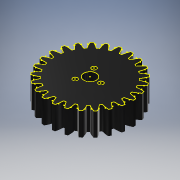
# Autodesk Inventor part: Spur Gear2
Saved by Autodesk Inventor 2017 (Build 210142000, 142)
## iProperties
Created: 2018-10-18
Part Number: Spur Gear2
Material: ABS Plastic
Document SubType Name: Modeling
Designer: Dell
Categories: <?xml version="1.0" encoding="UTF-16"?> <MemberInstance><Categories><FamilyTemplate><FamilyTemplateParameter ValueType="xs:double" Id="1" ObjectReferenceKey="da_z" ObjectType="kUserParameterObject"/><FamilyTemplateParameter ValueType="xs:double" Id="2" ObjectReferenceKey="da_b" ObjectType="kUserParameterObject"/><FamilyTemplateParameter ValueType="xs:double" Id="3" ObjectReferenceKey="da_beta" ObjectType="kUserParameterObject"/><FamilyTemplateParameter ValueType="xs:double" Id="4" ObjectReferenceKey="da_da" ObjectType="kUserParameterObject"/><FamilyTemplateParameter ValueType="xs:double" Id="5" ObjectReferenceKey="da_aw" ObjectType="kUserParameterObject"/><FamilyTemplateParameter ValueType="xs:string" Id="6" ObjectReferenceKey="EAIAABAAAACIAQAAAAAAAIAAAAAAAAAA" ObjectType="83910656" SubObjectId="SurfaceGeometry"/></FamilyTemplate><ParamToTemplateMap><ParamToTemplate CategoryParameter="//CategoryParameter[@InternalName='046C89C9-8512-4d59-83FE-43B91F4F132A']" TemplateParameter="1"/><ParamToTemplate CategoryParameter="//CategoryParameter[@InternalName='2552DF32-E462-4b46-AEBF-C6C7768E72AC']" TemplateParameter="2"/><ParamToTemplate CategoryParameter="//CategoryParameter[@InternalName='C9EE641D-15FC-4fae-A226-E94C4372FDD7']" TemplateParameter="3"/><ParamToTemplate><ParamToTemplate CategoryParameter="//CategoryParameter[@InternalName='00B6519A-459B-49c7-AD84-2E56D39A5744']" ConstantValue="0.000000"/></ParamToTemplate><ParamToTemplate><ParamToTemplate CategoryParameter="//CategoryParameter[@InternalName='04B31F0E-C7A6-4894-AA32-9629BEFACF47']" ConstantValue="1.000000"/></ParamToTemplate><ParamToTemplate><ParamToTemplate CategoryParameter="//CategoryParameter[@InternalName='43CBEC2E-7847-49e7-A936-2F7889FCB2D9']" ConstantValue="0.250000"/></ParamToTemplate><ParamToTemplate><ParamToTemplate CategoryParameter="//CategoryParameter[@InternalName='B1EFC894-105D-4ebd-86BF-FA20ED196853']" ConstantValue="0.350000"/></ParamToTemplate><ParamToTemplate><ParamToTemplate CategoryParameter="//CategoryParameter[@InternalName='51175063-3D10-4879-93E8-6246FE8B403D']" ConstantValue="2060000000.000000"/></ParamToTemplate><ParamToTemplate><ParamToTemplate CategoryParameter="//CategoryParameter[@InternalName='A3A52E27-4454-46a9-B0BD-C932399B70AF']" ConstantValue="0.300000"/></ParamToTemplate><ParamToTemplate><ParamToTemplate CategoryParameter="//CategoryParameter[@InternalName='91B76062-C214-41d9-B1B9-14D2AB99603D']" ConstantValue="0.200000"/></ParamToTemplate><ParamToTemplate><ParamToTemplate CategoryParameter="//CategoryParameter[@InternalName='374E806E-8B8A-4dda-A9AA-1039D6500AD2']" ConstantValue="5.000000"/></ParamToTemplate><ParamToTemplate><ParamToTemplate CategoryParameter="//CategoryParameter[@InternalName='2D373A89-B862-43d6-8D0B-0CBF12AB9F6C']" ConstantValue="0.349066"/></ParamToTemplate><ParamToTemplate CategoryParameter="//CategoryParameter[@InternalName='37777632-D6A2-4fac-9D53-DB8ACD95C989']" TemplateParameter="4"/><ParamToTemplate CategoryParameter="//CategoryParameter[@InternalName='FD1017F1-B727-4f7e-9707-0F86F1FF9423']" TemplateParameter="5"/><ParamToTemplate><ParamToTemplate CategoryParameter="//CategoryParameter[@InternalName='9E1B4470-B2D3-4ff1-B813-535BB4CDF51A']" ConstantValue="3520000.000000"/></ParamToTemplate><ParamToTemplate><ParamToTemplate CategoryParameter="//CategoryParameter[@InternalName='F8452263-BFF6-458c-9FB1-07C4B99E95CD']" ConstantValue="11400000.000000"/></ParamToTemplate><ParamToTemplate><ParamToTemplate CategoryParameter="//CategoryParameter[@InternalName='3E3BB259-FD49-497f-8171-6EBC954A3479']" ConstantValue="2.000000"/></ParamToTemplate><ParamToTemplate CategoryParameter="//CategoryParameter[@InternalName='27C3BAF2-7550-4e4b-AE2C-0DB134B7D9B7']" TemplateParameter="6"/></ParamToTemplateMap><Category DisplayName="Gear" InternalName="DC85795E-93AB-48d5-8EEE-5A27447B64BD" Mnemonic="Gear"><CategoryParameter DisplayName="z" InternalName="046C89C9-8512-4d59-83FE-43B91F4F132A" Mnemonic="z"/><CategoryParameter DisplayName="b" InternalName="2552DF32-E462-4b46-AEBF-C6C7768E72AC" Mnemonic="b"/><CategoryParameter DisplayName="||b|" InternalName="C9EE641D-15FC-4fae-A226-E94C4372FDD7" Mnemonic="beta"/><CategoryParameter DisplayName="x" InternalName="00B6519A-459B-49c7-AD84-2E56D39A5744" Mnemonic="x"/><CategoryParameter DisplayName="a*" InternalName="04B31F0E-C7A6-4894-AA32-9629BEFACF47" Mnemonic="a"/><CategoryParameter DisplayName="c*" InternalName="43CBEC2E-7847-49e7-A936-2F7889FCB2D9" Mnemonic="c"/><CategoryParameter DisplayName="r|.f|*" InternalName="B1EFC894-105D-4ebd-86BF-FA20ED196853" Mnemonic="rf"/><CategoryParameter DisplayName="E" InternalName="51175063-3D10-4879-93E8-6246FE8B403D" Mnemonic="E"/><CategoryParameter DisplayName="||m|" InternalName="A3A52E27-4454-46a9-B0BD-C932399B70AF" Mnemonic="mi"/><Category DisplayName="SpurGear" InternalName="26C5A22E-A91E-4dfd-A3B3-23CCAFAE1764" Mnemonic="SpurGear"><CategoryParameter DisplayName="m" InternalName="91B76062-C214-41d9-B1B9-14D2AB99603D" Mnemonic="m"/><CategoryParameter DisplayName="P" InternalName="374E806E-8B8A-4dda-A9AA-1039D6500AD2" Mnemonic="PP"/><CategoryParameter DisplayName="||a|" InternalName="2D373A89-B862-43d6-8D0B-0CBF12AB9F6C" Mnemonic="alpha"/><CategoryParameter DisplayName="d|.a|" InternalName="37777632-D6A2-4fac-9D53-DB8ACD95C989" Mnemonic="da"/><CategoryParameter DisplayName="a|.w|" InternalName="FD1017F1-B727-4f7e-9707-0F86F1FF9423" Mnemonic="aw"/><CategoryParameter DisplayName="||s||.Flim|" InternalName="9E1B4470-B2D3-4ff1-B813-535BB4CDF51A" Mnemonic="sFlim"/><CategoryParameter DisplayName="||s||.Hlim|" InternalName="F8452263-BFF6-458c-9FB1-07C4B99E95CD" Mnemonic="sHlim"/><CategoryParameter DisplayName="type" InternalName="3E3BB259-FD49-497f-8171-6EBC954A3479" Mnemonic="type"/><CategoryParameter DisplayName="PitchDiameter" InternalName="27C3BAF2-7550-4e4b-AE2C-0DB134B7D9B7" Mnemonic="IDS_PITCHDIAM"/></Category></Category></Categories></MemberInstance>
Density: 1.06 g/cm^3
Appearance: Smooth - Black
CustomPartVersion: 1
Author: Dell
Autodesk Inventor part; units mm, degrees
ref_plane "YZ Plane" through (0, 0, 0) normal (1, 0, 0) x (0, 1, 0)
ref_plane "XZ Plane" through (0, 0, 0) normal (0, 1, 0) x (-1, 0, 0)
ref_plane "XY Plane" through (0, 0, 0) normal (0, 0, 1) x (1, 0, 0)
sketch "Sketch1" plane through (0, 0, 0) normal (0, 0, 1) x (1, 0, 0)
  circle A0 centre (0, 0) radius 27
  dimension "d0" = 54
  constraints: 1 centre point
  measures "d0" diameter of A0
extrude "Extrusion1" add sketch "Sketch1" along normal blind 15
ref_plane "Work Plane2" through (0, 0, 7.5) normal (0, 0, 1) x (1, 0, 0)
sketch "Sketch2" plane through (0, 0, 0) normal (0, 0, -1) x (-1, 0, 0)
  circle A0 centre (0, 0) radius 27 projected
  circle A1 centre (0, 0) radius 25
  dimension "d3" = 50
  constraints: 1 centre point, 1 coincident
  measures "d3" diameter of A1
surface extrude "Pitch Diameter" sketch "Sketch2" against normal through all shown no curves A1
ref_plane "Work Plane8" through (0, 0, 0) normal (0.9921147, 0.1253332, 0) x (0, 0, 1)
ref_plane "Work Plane9" through (0, 0, 0) normal (1, 0, 0) x (0, 1, 0)
spur gear teeth "Spur Gear" teeth 25 pitch diameter 50 tip diameter 54 root diameter 45 face width 15 start plane through (0, 0, 0) normal (0, 0, -1) x (-1, 0, 0)
sketch "Sketch3" plane through (0, 0, 15) normal (0, 0, 1) x (1, 0, 0)
  circle A0 centre (0, 0) radius 4
  dimension "d49" = 8
  constraints: 1 centre point, 1 coincident
  measures "d49" diameter of A0
extrude "Extrusion2" cut sketch "Sketch3" against normal through all
sketch "Sketch4" plane through (0, 0, 0) normal (0, 0, -1) x (-1, 0, 0)
  circle A0 centre (0, 0) radius 12
  dimension "d52" = 24
  constraints: 1 centre point, 1 coincident
  measures "d52" diameter of A0
extrude "Extrusion3" cut sketch "Sketch4" against normal blind 6
sketch "Sketch5" plane through (0, 0, 15) normal (0, 0, 1) x (1, 0, 0)
  circle A0 centre (7, 0) radius 1.5
  circle A1 centre (-3.5, 6.0622) radius 1.5
  circle A2 centre (-3.5, -6.0622) radius 1.5
  point P0 (0, 0)
  dimension "d55" = 3
  dimension "d56" = 7
  dimension "d59" = 360
  constraints: 3 centre point, 1 horizontal alignment, 7 other
  measures "d55" diameter of A0
  measures "d56" distance of A0.centre point (0, 0)
extrude "Extrusion4" cut sketch "Sketch5" against normal through all
sketch "Sketch6" plane through (0, 0, 15) normal (0, 0, 1) x (1, 0, 0)
  circle A0 centre (-3.5, 6.0622) radius 1.5 projected
  circle A1 centre (7, 0) radius 1.5 projected
  circle A2 centre (-3.5, -6.0622) radius 1.5 projected
  circle A3 centre (0, 0) radius 4 projected
  arc A4 (-7.5328, 25.9279) -> (-7.6216, 21.1698) centre (10.7455, 23.2068) ccw projected
  arc A5 (-7.6216, 21.1698) -> (-8.9358, 20.6495) centre (0, 0) ccw projected
  arc A6 (-8.9358, 20.6495) -> (-12.2577, 24.0572) centre (-23.7193, 9.5612) ccw projected
  arc A7 (-12.2577, 24.0572) -> (-13.7441, 23.24) centre (0, 0) ccw projected
  arc A8 (-13.7441, 23.24) -> (-12.6469, 18.6093) centre (4.6367, 25.15) ccw projected
  arc A9 (-12.6469, 18.6093) -> (-13.7904, 17.7785) centre (0, 0) ccw projected
  arc A10 (-13.7904, 17.7785) -> (-17.8554, 20.253) centre (-25.3519, 3.3621) ccw projected
  arc A11 (-17.8554, 20.253) -> (-19.0919, 19.0919) centre (0, 0) ccw projected
  arc A12 (-19.0919, 19.0919) -> (-16.8775, 14.8795) centre (-1.7636, 25.5129) ccw projected
  arc A13 (-16.8775, 14.8795) -> (-17.7785, 13.7904) centre (0, 0) ccw projected
  arc A14 (-17.7785, 13.7904) -> (-22.3312, 15.1763) centre (-25.3915, -3.0483) ccw projected
  arc A15 (-22.3312, 15.1763) -> (-23.24, 13.7441) centre (0, 0) ccw projected
  arc A16 (-23.24, 13.7441) -> (-20.0476, 10.2148) centre (-8.053, 24.2728) ccw projected
  arc A17 (-20.0476, 10.2148) -> (-20.6495, 8.9358) centre (0, 0) ccw projected
  arc A18 (-20.6495, 8.9358) -> (-25.4038, 9.1459) centre (-23.8357, -9.2672) ccw projected
  arc A19 (-25.4038, 9.1459) -> (-25.9279, 7.5328) centre (0, 0) ccw projected
  arc A20 (-25.9279, 7.5328) -> (-21.9581, 4.9082) centre (-13.8364, 21.5075) ccw projected
  arc A21 (-21.9581, 4.9082) -> (-22.223, 3.5198) centre (0, 0) ccw projected
  arc A22 (-22.223, 3.5198) -> (-26.8802, 2.5409) centre (-20.7822, -14.9037) ccw projected
  arc A23 (-26.8802, 2.5409) -> (-26.9867, 0.8481) centre (0, 0) ccw projected
  arc A24 (-26.9867, 0.8481) -> (-22.4889, -0.7067) centre (-18.7504, 17.3909) ccw projected
  arc A25 (-22.4889, -0.7067) -> (-22.4001, -2.1174) centre (0, 0) ccw projected
  arc A26 (-22.4001, -2.1174) -> (-26.6676, -4.2237) centre (-16.4229, -19.6038) ccw projected
  arc A27 (-26.6676, -4.2237) -> (-26.3498, -5.8899) centre (0, 0) ccw projected
  arc A28 (-26.3498, -5.8899) -> (-21.6066, -6.2773) centre (-22.4862, 12.1815) ccw projected
  arc A29 (-21.6066, -6.2773) -> (-21.1698, -7.6216) centre (0, 0) ccw projected
  arc A30 (-21.1698, -7.6216) -> (-24.7794, -10.723) centre (-11.0317, -23.0721) ccw projected
  arc A31 (-24.7794, -10.723) -> (-24.0572, -12.2577) centre (0, 0) ccw projected
  arc A32 (-24.0572, -12.2577) -> (-19.3667, -11.4534) centre (-24.8092, 6.2067) ccw projected
  arc A33 (-19.3667, -11.4534) -> (-18.6093, -12.6469) centre (0, 0) ccw projected
  arc A34 (-18.6093, -12.6469) -> (-21.3342, -16.5485) centre (-4.9473, -25.0907) ccw projected
  arc A35 (-21.3342, -16.5485) -> (-20.253, -17.8554) centre (0, 0) ccw projected
  arc A36 (-20.253, -17.8554) -> (-15.9099, -15.9099) centre (-25.5733, -0.1581) ccw projected
  arc A37 (-15.9099, -15.9099) -> (-14.8795, -16.8775) centre (0, 0) ccw projected
  arc A38 (-14.8795, -16.8775) -> (-16.5485, -21.3342) centre (1.448, -25.5328) ccw projected
  arc A39 (-16.5485, -21.3342) -> (-15.1763, -22.3312) centre (0, 0) ccw projected
  arc A40 (-15.1763, -22.3312) -> (-11.4534, -19.3667) centre (-24.7306, -6.513) ccw projected
  arc A41 (-11.4534, -19.3667) -> (-10.2148, -20.0476) centre (0, 0) ccw projected
  arc A42 (-10.2148, -20.0476) -> (-10.723, -24.7794) centre (7.7522, -24.3705) ccw projected
  arc A43 (-10.723, -24.7794) -> (-9.1459, -25.4038) centre (0, 0) ccw projected
  arc A44 (-9.1459, -25.4038) -> (-6.2773, -21.6066) centre (-22.3339, -12.4586) ccw projected
  arc A45 (-6.2773, -21.6066) -> (-4.9082, -21.9581) centre (0, 0) ccw projected
  arc A46 (-4.9082, -21.9581) -> (-4.2237, -26.6676) centre (13.5694, -21.677) ccw projected
  arc A47 (-4.2237, -26.6676) -> (-2.5409, -26.8802) centre (0, 0) ccw projected
  arc A48 (-2.5409, -26.8802) -> (-0.7067, -22.4889) centre (-18.5339, -17.6214) ccw projected
  arc A49 (-0.7067, -22.4889) -> (0.7067, -22.4889) centre (0, 0) ccw projected
  arc A50 (0.7067, -22.4889) -> (2.5409, -26.8802) centre (18.5339, -17.6214) ccw projected
  arc A51 (2.5409, -26.8802) -> (4.2237, -26.6676) centre (0, 0) ccw projected
  arc A52 (4.2237, -26.6676) -> (4.9082, -21.9581) centre (-13.5694, -21.677) ccw projected
  arc A53 (4.9082, -21.9581) -> (6.2773, -21.6066) centre (0, 0) ccw projected
  arc A54 (6.2773, -21.6066) -> (9.1459, -25.4038) centre (22.3339, -12.4586) ccw projected
  arc A55 (9.1459, -25.4038) -> (10.723, -24.7794) centre (0, 0) ccw projected
  arc A56 (10.723, -24.7794) -> (10.2148, -20.0476) centre (-7.7522, -24.3705) ccw projected
  arc A57 (10.2148, -20.0476) -> (11.4534, -19.3667) centre (0, 0) ccw projected
  arc A58 (11.4534, -19.3667) -> (15.1763, -22.3312) centre (24.7306, -6.513) ccw projected
  arc A59 (15.1763, -22.3312) -> (16.5485, -21.3342) centre (0, 0) ccw projected
  arc A60 (16.5485, -21.3342) -> (14.8795, -16.8775) centre (-1.448, -25.5328) ccw projected
  arc A61 (14.8795, -16.8775) -> (15.9099, -15.9099) centre (0, 0) ccw projected
  arc A62 (15.9099, -15.9099) -> (20.253, -17.8554) centre (25.5733, -0.1581) ccw projected
  arc A63 (20.253, -17.8554) -> (21.3342, -16.5485) centre (0, 0) ccw projected
  arc A64 (21.3342, -16.5485) -> (18.6093, -12.6469) centre (4.9473, -25.0907) ccw projected
  arc A65 (18.6093, -12.6469) -> (19.3667, -11.4534) centre (0, 0) ccw projected
  arc A66 (19.3667, -11.4534) -> (24.0572, -12.2577) centre (24.8092, 6.2067) ccw projected
  arc A67 (24.0572, -12.2577) -> (24.7794, -10.723) centre (0, 0) ccw projected
  arc A68 (24.7794, -10.723) -> (21.1698, -7.6216) centre (11.0317, -23.0721) ccw projected
  arc A69 (21.1698, -7.6216) -> (21.6066, -6.2773) centre (0, 0) ccw projected
  arc A70 (21.6066, -6.2773) -> (26.3498, -5.8899) centre (22.4862, 12.1815) ccw projected
  arc A71 (26.3498, -5.8899) -> (26.6676, -4.2237) centre (0, 0) ccw projected
  arc A72 (26.6676, -4.2237) -> (22.4001, -2.1174) centre (16.4229, -19.6038) ccw projected
  arc A73 (22.4001, -2.1174) -> (22.4889, -0.7067) centre (0, 0) ccw projected
  arc A74 (22.4889, -0.7067) -> (26.9867, 0.8481) centre (18.7504, 17.3909) ccw projected
  arc A75 (26.9867, 0.8481) -> (26.8802, 2.5409) centre (0, 0) ccw projected
  arc A76 (26.8802, 2.5409) -> (22.223, 3.5198) centre (20.7822, -14.9037) ccw projected
  arc A77 (22.223, 3.5198) -> (21.9581, 4.9082) centre (0, 0) ccw projected
  arc A78 (21.9581, 4.9082) -> (25.9279, 7.5328) centre (13.8364, 21.5075) ccw projected
  arc A79 (25.9279, 7.5328) -> (25.4038, 9.1459) centre (0, 0) ccw projected
  arc A80 (25.4038, 9.1459) -> (20.6495, 8.9358) centre (23.8357, -9.2672) ccw projected
  arc A81 (20.6495, 8.9358) -> (20.0476, 10.2148) centre (0, 0) ccw projected
  arc A82 (20.0476, 10.2148) -> (23.24, 13.7441) centre (8.053, 24.2728) ccw projected
  arc A83 (23.24, 13.7441) -> (22.3312, 15.1763) centre (0, 0) ccw projected
  arc A84 (22.3312, 15.1763) -> (17.7785, 13.7904) centre (25.3915, -3.0483) ccw projected
  arc A85 (17.7785, 13.7904) -> (16.8775, 14.8795) centre (0, 0) ccw projected
  arc A86 (16.8775, 14.8795) -> (19.0919, 19.0919) centre (1.7636, 25.5129) ccw projected
  arc A87 (19.0919, 19.0919) -> (17.8554, 20.253) centre (0, 0) ccw projected
  arc A88 (17.8554, 20.253) -> (13.7904, 17.7785) centre (25.3519, 3.3621) ccw projected
  arc A89 (13.7904, 17.7785) -> (12.6469, 18.6093) centre (0, 0) ccw projected
  arc A90 (12.6469, 18.6093) -> (13.7441, 23.24) centre (-4.6367, 25.15) ccw projected
  arc A91 (13.7441, 23.24) -> (12.2577, 24.0572) centre (0, 0) ccw projected
  arc A92 (12.2577, 24.0572) -> (8.9358, 20.6495) centre (23.7193, 9.5612) ccw projected
  arc A93 (8.9358, 20.6495) -> (7.6216, 21.1698) centre (0, 0) ccw projected
  arc A94 (7.6216, 21.1698) -> (7.5328, 25.9279) centre (-10.7455, 23.2068) ccw projected
  arc A95 (7.5328, 25.9279) -> (5.8899, 26.3498) centre (0, 0) ccw projected
  arc A96 (5.8899, 26.3498) -> (3.5198, 22.223) centre (20.5963, 15.1595) ccw projected
  arc A97 (3.5198, 22.223) -> (2.1174, 22.4001) centre (0, 0) ccw projected
  arc A98 (2.1174, 22.4001) -> (0.8481, 26.9867) centre (-16.1792, 19.8054) ccw projected
  arc A99 (0.8481, 26.9867) -> (-0.8481, 26.9867) centre (0, 0) ccw projected
  arc A100 (-0.8481, 26.9867) -> (-2.1174, 22.4001) centre (16.1792, 19.8054) ccw projected
  arc A101 (-2.1174, 22.4001) -> (-3.5198, 22.223) centre (0, 0) ccw projected
  arc A102 (-3.5198, 22.223) -> (-5.8899, 26.3498) centre (-20.5963, 15.1595) ccw projected
  arc A103 (-5.8899, 26.3498) -> (-7.5328, 25.9279) centre (0, 0) ccw projected
equation "\"d0\" = da_da"
equation "\"d1\" = da_b"
equation "\"d3\" = da_dw"
equation "\"d50\" = d49"
equation "\"da_da\" = 54"
equation "\"da_b\" = 15"
equation "\"da_dw\" = 50"
body "Solid1"
body "Srf1"
